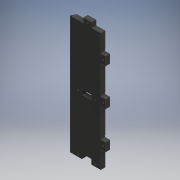
# Autodesk Inventor part: BA03
Saved by Autodesk Inventor 2017 (Build 210142000, 142)
## iProperties
Created: 2019-05-22
Part Number: BA03
Material: Wood (Cherry)
Document SubType Name: Modeling
Designer: Dell
Density: 0.63 g/cm^3
Appearance: Smooth - Black
Mass: 235.193 g
Surface Area: 754.585 cm^2
Volume: 373.322 cm^3
Author: Dell
Autodesk Inventor part; units mm, degrees
ref_plane "YZ Plane" through (0, 0, 0) normal (1, 0, 0) x (0, 1, 0)
ref_plane "XZ Plane" through (0, 0, 0) normal (0, 1, 0) x (-1, 0, 0)
ref_plane "XY Plane" through (0, 0, 0) normal (0, 0, 1) x (1, 0, 0)
sketch "Sketch1" plane through (0, 0, 0) normal (0, 0, 1) x (1, 0, 0)
  line L0 (0, 0) -> (88.9, 0)
  line L1 (88.9, 0) -> (88.9, 12.7)
  line L2 (88.9, 12.7) -> (7.3323, 12.7)
  line L3 (7.3323, 12.7) -> (0, 0)
  dimension "d0" = 88.9
  dimension "d1" = 12.7
  dimension "d2" = 60
  constraints: 8 end point, 2 perpendicular, 1 horizontal
  measures "d0" distance of L0.start L0.end
  measures "d1" distance of L0.end L1.end
  measures "d2" angle of L0 L3
extrude "Extrusion1" add sketch "Sketch1" along normal blind 342.9
sketch "Sketch2" plane through (0, 0, 0) normal (0, -1, 0) x (1, 0, 0)
  line L0 (38.1, 342.9) -> (63.5, 342.9)
  line L1 (63.5, 342.9) -> (63.5, 355.6)
  line L2 (63.5, 355.6) -> (38.1, 355.6)
  line L3 (38.1, 355.6) -> (38.1, 342.9)
  line L4 (0, 342.9) -> (101.6, 342.9)
  line L5 (0, 342.9) -> (88.9, 342.9) projected
  point P0 (0, 0)
  point P1 (50.8, 342.9)
  dimension "d5" = 25.4
  dimension "d6" = 12.7
  dimension "d9" = 101.6
  constraints: 10 end point, 2 midpoint, 2 parallel, 1 collinear, 1 horizontal, 1 perpendicular
  measures "d5" distance of L2.end L1.end
  measures "d6" distance of L1.end L0.end
  measures "d9" distance of L4.start L4.end
extrude "Extrusion2" add sketch "Sketch2" against normal blind 12.7
sketch "Sketch3" plane through (0, 0, 0) normal (0, -1, 0) x (1, 0, 0)
  line L0 (63.5, 342.9) -> (63.5, 355.6) projected
  line L1 (63.5, 355.6) -> (38.1, 355.6) projected
  circle A0 centre (50.8, 349.25) radius 2.25
  point P0 (0, 0)
  point P1 (50.8, 355.6)
  point P2 (63.5, 349.25)
  dimension "d10" = 4.5
  constraints: 2 midpoint, 1 centre point, 1 horizontal alignment, 1 vertical alignment
  measures "d10" diameter of A0
extrude "Extrusion3" cut sketch "Sketch3" against normal through all
sketch "Sketch4" plane through (0, 0, 0) normal (0, -1, 0) x (1, 0, 0)
  line L0 (88.9, 0) -> (88.9, 342.9) projected
  line L1 (88.9, 50.8) -> (101.6, 50.8)
  line L2 (101.6, 50.8) -> (101.6, 76.2)
  line L3 (101.6, 76.2) -> (88.9, 76.2)
  line L4 (88.9, 76.2) -> (88.9, 50.8)
  line L5 (88.9, 292.1) -> (101.6, 292.1)
  line L6 (101.6, 292.1) -> (101.6, 266.7)
  line L7 (101.6, 266.7) -> (88.9, 266.7)
  line L8 (88.9, 266.7) -> (88.9, 292.1)
  line L9 (88.9, 184.15) -> (101.6, 184.15)
  line L10 (101.6, 184.15) -> (101.6, 158.75)
  line L11 (101.6, 158.75) -> (88.9, 158.75)
  line L12 (88.9, 158.75) -> (88.9, 184.15)
  circle A0 centre (95.25, 279.4) radius 2.25
  circle A1 centre (95.25, 171.45) radius 2.25
  circle A2 centre (95.25, 63.5) radius 2.25
  point P0 (0, 0)
  point P1 (88.9, 171.45)
  point P2 (95.25, 292.1)
  point P3 (95.25, 184.15)
  point P4 (95.25, 76.2)
  point P5 (101.6, 279.4)
  point P6 (101.6, 171.45)
  point P7 (101.6, 63.5)
  dimension "d14" = 25.4
  dimension "d15" = 12.7
  dimension "d16" = 25.4
  dimension "d18" = 25.4
  dimension "d19" = 50.8
  dimension "d20" = 50.8
  dimension "d21" = 4.5
  dimension "d22" = 4.5
  dimension "d23" = 4.5
  constraints: 24 end point, 8 midpoint, 6 parallel, 5 vertical alignment, 3 centre point, 3 horizontal, 3 horizontal alignment, 3 perpendicular, 3 point on line
  measures "d14" distance of L2.end L1.end
  measures "d15" distance of L6.end L7.end
  measures "d16" distance of L5.end L6.end
  measures "d18" distance of L9.end L10.end
  measures "d19" distance from line of L0.end L5
  measures "d20" distance from line of L0.start L1
  measures "d21" diameter of A0
  measures "d22" diameter of A1
  measures "d23" diameter of A2
extrude "Extrusion4" add sketch "Sketch4" against normal blind 12.7
sketch "Sketch6" plane through (88.9, 0, 292.1) normal (0, 0, 1) x (1, 0, 0)
  line L0 (-88.9, 0) -> (-66.903, 12.7)
  line L1 (0, 12.7) -> (-81.5677, 12.7) projected
  line L2 (-88.9, 0) -> (0, 0) projected
  line L3 (-66.903, 12.7) -> (-66.903, 0)
  line L4 (-81.5677, 12.7) -> (-88.9, 0) projected
  line L5 (-77.9015, 6.35) -> (-77.9015, 12.7)
  line L6 (-77.9015, 12.7) -> (-81.5677, 12.7)
  dimension "d28" = 30
  dimension "d31" = 12.7
  constraints: 8 end point, 3 point on line, 1 collinear, 1 midpoint, 1 perpendicular, 1 vertical
  measures "d28" angle of L0 L2
  measures "d31" distance of L0.start L5.start
extrude "Extrusion6" [suppressed]
sketch "Sketch7" plane through (88.9, 0, 184.15) normal (0, 0, 1) x (1, 0, 0)
  line L0 (-77.9015, 12.7) -> (-77.9015, 6.35) projected
  line L1 (-81.5677, 12.7) -> (-77.9015, 12.7) projected
  line L2 (-88.9, 0) -> (-81.5677, 12.7) projected
  line L3 (-77.9015, 6.35) -> (-88.9, 0) projected
  point P0 (-88.9, 0)
extrude "Extrusion7" [suppressed]
sketch "Sketch8" plane through (88.9, 0, 76.2) normal (0, 0, 1) x (1, 0, 0)
  line L0 (-77.9015, 12.7) -> (-77.9015, 6.35) projected
  line L1 (-81.5677, 12.7) -> (-77.9015, 12.7) projected
  line L2 (-88.9, 0) -> (-81.5677, 12.7) projected
  line L3 (-77.9015, 6.35) -> (-88.9, 0) projected
  point P0 (-88.9, 0)
extrude "Extrusion8" [suppressed]
sketch "Sketch10" plane through (7.3323, 12.7, 0) normal (0, 1, 0) x (1, 0, 0)
  circle A0 centre (15.7838, -6.35) radius 2.25
  line L0 (80.6319, -12.7) -> (0.9358, -12.7)
  circle A1 centre (65.7838, -6.35) radius 2.25
  line L1 (28.0838, -12.7) -> (53.4838, -12.7)
  line L2 (53.4838, -12.7) -> (53.4838, 0)
  line L3 (53.4838, 0) -> (28.0838, 0)
  line L4 (28.0838, 0) -> (28.0838, -12.7)
  line L5 (15.7838, -6.35) -> (65.7838, -6.35) construction
  line L6 (81.5677, 0) -> (0, 0) projected
  point P0 (-7.3323, 0)
  point P1 (40.7838, -6.35)
  point P2 (40.7838, -12.7)
  point P3 (40.7838, -12.7)
  point P4 (40.7838, 0)
  point P5 (28.0838, -6.35)
  dimension "d39" = 4.5
  dimension "d41" = 4.5
  dimension "d42" = 25.4
  dimension "d43" = 12.7
  dimension "d44" = 50
  constraints: 12 end point, 8 midpoint, 3 horizontal, 2 centre point, 2 parallel, 1 horizontal alignment, 1 perpendicular, 1 point on line, 1 vertical alignment
  measures "d39" diameter of A0
  measures "d41" diameter of A1
  measures "d42" distance of L3.end L2.end
  measures "d43" distance of L2.end L1.end
  measures "d44" distance of L5.start L5.end
extrude "Extrusion10" cut sketch "Sketch10" against normal through all
sketch "Sketch11" plane through (38.1, 0, 355.6) normal (0, -1, 0) x (1, 0, 0)
  line L0 (22.7162, -194.15) -> (-2.6838, -194.15)
  line L1 (-2.6838, -194.15) -> (-2.6838, -181.45)
  line L2 (-2.6838, -181.45) -> (22.7162, -181.45)
  line L3 (22.7162, -181.45) -> (22.7162, -194.15)
  line L4 (63.5, -171.45) -> (50.8, -171.45) projected
  line L5 (-2.6838, -342.9) -> (22.7162, -342.9) projected
  point P0 (-38.1, -355.6)
  point P1 (10.0162, -194.15)
  point P2 (10.0162, -342.9)
  dimension "d47" = 25.4
  dimension "d48" = 12.7
  dimension "d85" = 10
  constraints: 8 end point, 2 midpoint, 2 parallel, 1 horizontal, 1 perpendicular, 1 vertical alignment
  measures "d47" distance of L1.end L2.end
  measures "d48" distance of L0.end L1.end
  measures "d85" vertical distance of L2.end L4.start
extrude "Extrusion11" cut sketch "Sketch11" against normal through all
sketch "Sketch12" plane through (38.1, 0, 355.6) normal (0, -1, 0) x (1, 0, 0)
  circle A0 centre (-14.9838, -187.8) radius 2.25
  circle A1 centre (35.0162, -187.8) radius 2.25
  circle A2 centre (-14.9838, -349.25) radius 2.25 projected
  circle A3 centre (35.0162, -349.25) radius 2.25 projected
  line L0 (22.7162, -181.45) -> (22.7162, -194.15) projected
  point P0 (-38.1, -355.6)
  point P1 (22.7162, -187.8)
  dimension "d52" = 4.5
  dimension "d53" = 4.5
  constraints: 2 centre point, 2 horizontal alignment, 2 vertical alignment, 1 midpoint
  measures "d52" diameter of A0
  measures "d53" diameter of A1
extrude "Extrusion12" cut sketch "Sketch12" against normal through all contours A0 | A1
sketch "Sketch13" plane through (7.3323, 12.7, 342.9) normal (0, 1, 0) x (1, 0, 0)
  line L0 (53.4838, 342.9) -> (81.5677, 342.9) projected
  line L1 (54.7538, 342.9) -> (26.8138, 342.9)
  line L2 (26.8138, 342.9) -> (26.8138, 328.93)
  line L3 (26.8138, 328.93) -> (54.7538, 328.93)
  line L4 (54.7538, 328.93) -> (54.7538, 342.9)
  line L5 (54.7538, 182.72) -> (26.8138, 182.72)
  line L6 (26.8138, 182.72) -> (26.8138, 167.48)
  line L7 (26.8138, 167.48) -> (54.7538, 167.48)
  line L8 (54.7538, 167.48) -> (54.7538, 182.72)
  line L9 (53.4838, 330.2) -> (28.0838, 330.2) projected
  line L10 (28.0838, 181.45) -> (53.4838, 181.45) projected
  line L11 (53.4838, 181.45) -> (53.4838, 168.75) projected
  circle A0 centre (58.4127, -2.2451) radius 3.175
  circle A1 centre (28.5226, -2.2451) radius 3.175
  circle A2 centre (83.8127, 48.5549) radius 3.175
  circle A3 centre (83.8127, 78.4451) radius 3.175
  circle A4 centre (83.8127, 156.5049) radius 3.175
  circle A5 centre (83.8127, 186.3951) radius 3.175
  circle A6 centre (83.8127, 264.4549) radius 3.175
  circle A7 centre (83.8127, 294.3451) radius 3.175
  line L12 (94.2677, 292.1) -> (81.5677, 292.1) projected
  line L13 (81.5677, 292.1) -> (83.8127, 294.3451)
  line L14 (58.4127, -2.2451) -> (56.1677, 0) construction
  line L15 (56.1677, -12.7) -> (56.1677, 0) projected
  point P0 (-7.3323, 342.9)
  point P1 (40.7838, 330.2)
  point P2 (40.7838, 328.93)
  point P3 (40.7838, 181.45)
  point P4 (40.7838, 182.72)
  point P5 (53.4838, 175.1)
  point P6 (54.7538, 175.1)
  point P7 (81.5677, 266.7)
  point P8 (81.5677, 184.15)
  point P9 (81.5677, 158.75)
  point P10 (81.5677, 50.8)
  point P11 (81.5677, 76.2)
  point P12 (30.7677, 0)
  dimension "d61" = 6.35
  dimension "d62" = 6.35
  dimension "d63" = 6.35
  dimension "d64" = 6.35
  dimension "d65" = 6.35
  dimension "d66" = 6.35
  dimension "d67" = 6.35
  dimension "d68" = 6.35
  dimension "d56" = 1.27
  dimension "d57" = 1.27
  dimension "d58" = 1.27
  dimension "d69" = 45
  dimension "d70" = 45
  constraints: 20 end point, 9 vertical alignment, 6 midpoint, 4 parallel, 3 point on line, 2 horizontal, 2 horizontal alignment, 2 perpendicular, 1 coincident, 24 other
  measures "d56" distance between parallel lines of L3 L9
  measures "d57" distance between parallel lines of L8 L11
  measures "d58" distance between parallel lines of L5 L10
  measures "d69" angle of L12 L13
  measures "d70" angle of L15 L14
extrude "Extrusion13" cut sketch "Sketch13" against normal through all
sketch "Sketch14" plane through (7.3323, 12.7, 342.9) normal (0, 1, 0) x (1, 0, 0)
  line L0 (94.2677, 50.8) -> (86.0578, 50.8) projected
  line L1 (94.2677, 50.8) -> (85.1491, 50.8)
  line L2 (85.1491, 50.8) -> (85.1491, 51.435)
  line L3 (85.1491, 51.435) -> (94.2677, 51.435)
  line L4 (94.2677, 51.435) -> (94.2677, 50.8)
  line L5 (94.2677, 50.8) -> (94.2677, 76.2) projected
  line L6 (94.2677, 76.2) -> (85.1491, 76.2)
  line L7 (85.1491, 76.2) -> (85.1491, 75.565)
  line L8 (85.1491, 75.565) -> (94.2677, 75.565)
  line L9 (94.2677, 75.565) -> (94.2677, 76.2)
  line L10 (94.2677, 158.75) -> (86.0578, 158.75) projected
  line L11 (94.2677, 158.75) -> (85.1491, 158.75)
  line L12 (85.1491, 158.75) -> (85.1491, 159.385)
  line L13 (85.1491, 159.385) -> (94.2677, 159.385)
  line L14 (94.2677, 159.385) -> (94.2677, 158.75)
  line L15 (86.0578, 184.15) -> (94.2677, 184.15) projected
  line L16 (94.2677, 184.15) -> (85.1491, 184.15)
  line L17 (85.1491, 184.15) -> (85.1491, 183.515)
  line L18 (85.1491, 183.515) -> (94.2677, 183.515)
  line L19 (94.2677, 183.515) -> (94.2677, 184.15)
  line L20 (94.2677, 266.7) -> (94.2677, 292.1) projected
  line L21 (94.2677, 266.7) -> (85.1491, 266.7)
  line L22 (85.1491, 266.7) -> (85.1491, 267.335)
  line L23 (85.1491, 267.335) -> (94.2677, 267.335)
  line L24 (94.2677, 267.335) -> (94.2677, 266.7)
  line L25 (94.2677, 292.1) -> (85.1491, 292.1)
  line L26 (85.1491, 292.1) -> (85.1491, 291.465)
  line L27 (85.1491, 291.465) -> (94.2677, 291.465)
  line L28 (94.2677, 291.465) -> (94.2677, 292.1)
  arc A0 (81.5677, 296.5901) -> (86.0578, 292.1) centre (83.8127, 294.3451) ccw projected
  line L29 (30.7677, -12.7) -> (56.1677, -12.7) projected
  arc A1 (60.6578, 0) -> (56.1677, -4.4901) centre (58.4127, -2.2451) ccw projected
  line L30 (56.1677, -12.7) -> (55.5327, -12.7)
  line L31 (55.5327, -12.7) -> (55.5327, -3.5814)
  line L32 (55.5327, -3.5814) -> (56.1677, -3.5814)
  line L33 (56.1677, -3.5814) -> (56.1677, -12.7)
  line L34 (30.7677, -4.4901) -> (30.7677, -12.7) projected
  arc A2 (30.7677, -4.4901) -> (26.2775, 0) centre (28.5226, -2.2451) ccw projected
  line L35 (30.7677, -12.7) -> (31.4027, -12.7)
  line L36 (31.4027, -12.7) -> (31.4027, -3.5814)
  line L37 (31.4027, -3.5814) -> (30.7677, -3.5814)
  line L38 (30.7677, -3.5814) -> (30.7677, -12.7)
  point P0 (-7.3323, 342.9)
  dimension "d71" = 0.635
  dimension "d72" = 0.635
  dimension "d73" = 0.635
  dimension "d74" = 0.635
  dimension "d75" = 0.635
  dimension "d76" = 0.635
  dimension "d77" = 0.635
  constraints: 64 end point, 16 parallel, 8 horizontal, 8 perpendicular, 5 point on line, 3 point on circle, 1 vertical alignment
  measures "d71" distance between parallel lines of L25 L27
  measures "d72" distance between parallel lines of L21 L23
  measures "d73" distance between parallel lines of L16 L18
  measures "d74" distance between parallel lines of L11 L13
  measures "d75" distance between parallel lines of L0 L3
  measures "d76" distance between parallel lines of L6 L8
  measures "d77" distance between parallel lines of L33 L31
extrude "Extrusion14" cut sketch "Sketch14" against normal through all
sketch "Sketch15" plane through (7.3323, 12.7, 342.9) normal (0, 1, 0) x (1, 0, 0)
  line L0 (94.2677, 267.335) -> (85.1491, 267.335) projected
  line L1 (94.2677, 267.335) -> (95.5377, 267.335)
  line L2 (95.5377, 267.335) -> (95.5377, 291.465)
  line L3 (95.5377, 291.465) -> (94.2677, 291.465)
  line L4 (94.2677, 291.465) -> (94.2677, 267.335)
  line L5 (94.2677, 183.515) -> (95.5377, 183.515)
  line L6 (95.5377, 183.515) -> (95.5377, 159.385)
  line L7 (95.5377, 159.385) -> (94.2677, 159.385)
  line L8 (94.2677, 159.385) -> (94.2677, 183.515)
  line L9 (94.2677, 51.435) -> (94.2677, 75.565) projected
  line L10 (94.2677, 75.565) -> (95.5377, 75.565)
  line L11 (95.5377, 75.565) -> (95.5377, 51.435)
  line L12 (95.5377, 51.435) -> (94.2677, 51.435)
  line L13 (94.2677, 51.435) -> (94.2677, 75.565)
  line L14 (31.4027, -12.7) -> (55.5327, -12.7) projected
  line L15 (55.5327, -12.7) -> (31.4027, -12.7)
  line L16 (31.4027, -12.7) -> (31.4027, -13.97)
  line L17 (31.4027, -13.97) -> (55.5327, -13.97)
  line L18 (55.5327, -13.97) -> (55.5327, -12.7)
  point P0 (-7.3323, 342.9)
  dimension "d80" = 1.27
  dimension "d81" = 1.27
  constraints: 32 end point, 8 parallel, 4 horizontal, 4 perpendicular, 3 coincident, 2 point on line, 1 vertical alignment
  measures "d80" distance of L2.end point (94.268, 291.465)
  measures "d81" distance of L17.end L14.end
extrude "Extrusion15" add sketch "Sketch15" against normal blind 12.7
equation "\"d1\" = Panel_Thickness"
equation "\"d6\" = Panel_Thickness"
equation "\"d7\" = Panel_Thickness"
equation "\"d15\" = Panel_Thickness"
equation "\"d24\" = Panel_Thickness"
equation "\"d43\" = Panel_Thickness"
equation "\"d48\" = Panel_Thickness"
equation "\"d61\" = d63"
equation "\"d62\" = d61"
equation "\"d63\" = d65"
equation "\"d64\" = d65"
equation "\"d65\" = d68"
equation "\"d66\" = d68"
equation "\"d67\" = d68"
equation "\"d68\" = Tool_Dia"
equation "\"d56\" = Fit_Tolerance"
equation "\"d57\" = Fit_Tolerance"
equation "\"d58\" = Fit_Tolerance"
equation "\"d71\" = 0.5 * Fit_Tolerance"
equation "\"d72\" = 0.5 * Fit_Tolerance"
equation "\"d73\" = 0.5 * Fit_Tolerance"
equation "\"d74\" = 0.5 * Fit_Tolerance"
equation "\"d75\" = 0.5 * Fit_Tolerance"
equation "\"d76\" = 0.5 * Fit_Tolerance"
equation "\"d77\" = 0.5 * Fit_Tolerance"
equation "\"d80\" = Fit_Tolerance"
equation "\"d81\" = Fit_Tolerance"
equation "\"d82\" = Panel_Thickness"
equation "\"Panel_Thickness\" = 12.7"
equation "\"Fit_Tolerance\" = 1.27"
equation "\"Tool_Dia\" = 6.35"
body "Solid1"
